Autodesk Inventor part; units mm, degrees
(part 2 of 2)
extrude "押し出し17" cut sketch "スケッチ5" against normal blind 1.5 contours A36 L272 | L272 A36
extrude "押し出し18" cut sketch "スケッチ5" against normal blind 1.5 contours A38 L274 | L274 A38
extrude "押し出し19" cut sketch "スケッチ5" against normal blind 1.5 contours L265 L269 L268 L267
extrude "押し出し20" cut sketch "スケッチ5" against normal blind 1.5 contours L290 L291 L292 L238
fillet "フィレット1" radius 0.8 4 edges at (-19, 8.5, -0.5) (-19, -8.5, -0.5) (19, -8.5, -0.5) (19, 8.5, -0.5)
fillet "フィレット2" radius 0.8 26 edges at (-26, 15.5, -0.5) (-24, 13.5, -0.5) (-20.8255, 13.5, -0.5) (-15.3255, 19, -0.5) (15.3255, 19, -0.5) (20.8255, 13.5, -0.5) (24, 13.5, -0.5) (26, 15.5, -0.5) (26, 24.1685, -0.5) (21.8107, 27.6837, -0.5) (-26, 24.1685, -0.5) (-21.8107, 27.6837, -0.5) (-18.1736, 44.795, -0.5) (-4.6137, 54.2897, -0.5) (4.6137, 54.2897, -0.5) (18.1736, 44.795, -0.5) (-23.55, -14.1999, -0.5) (-23.2643, -13.5, -0.5) (-21.2643, -13.5, -0.5) (-11.6308, -20, -0.5) (-11.5077, -26, -0.5) (11.5077, -26, -0.5) (11.6308, -20, -0.5) (21.2643, -13.5, -0.5) (23.55, -14.1999, -0.5) (23.2643, -13.5, -0.5)
fillet "フィレット3" radius 0.8 28 edges at (-6.6203, -29.5, -0.5) (-8.1203, -31, -0.5) (-12.1203, -31, -0.5) (6.6203, -29.5, -0.5) (8.1203, -31, -0.5) (12.1203, -31, -0.5) (31, -12.5, -0.5) (31, -9.3, -0.5) (30.2, -8.5, -0.5) (29, 8.5, -0.5) (31, 10.5, -0.5) (31, 26.5, -0.5) (26.3435, 30.4073, -0.5) (22.0451, 50.6295, -0.5) (9.6771, 59.2897, -0.5) (3.6771, 59.2897, -0.5) (0.9296, 58.2897, -0.5) (-0.9296, 58.2897, -0.5) (-3.6771, 59.2897, -0.5) (-9.6771, 59.2897, -0.5) (-22.0451, 50.6295, -0.5) (-26.3435, 30.4073, -0.5) (-31, 26.5, -0.5) (-31, 10.5, -0.5) (-29, 8.5, -0.5) (-30.2, -8.5, -0.5) (-31, -9.3, -0.5) (-31, -12.5, -0.5)
extrude "押し出し23" cut sketch "スケッチ5" against normal blind 1 contours A41 | A42
